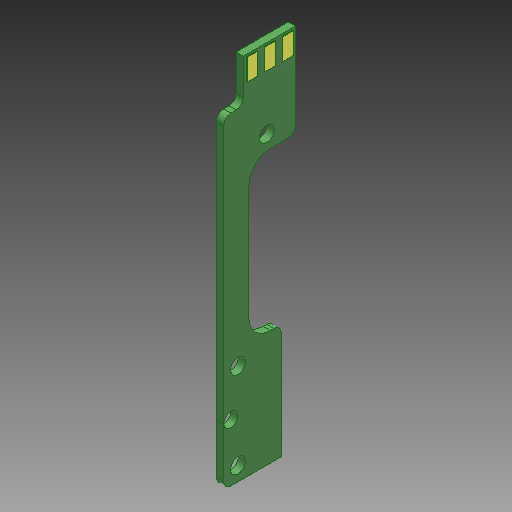
# Autodesk Inventor part: IR Platine
Saved by Autodesk Inventor 2019.1 (Build 231200000, 200)
## iProperties
Part Number: IR Platine
Material: Phenolharz
Document SubType Name: Modeling
Designer: rYan
Mass: 0.429024 g
Surface Area: 7.74127 cm^2
Volume: 0.310887 cm^3
Density: 1.38 g/cm^3
Appearance: Glatt - waldgrün
Author: rYan
Autodesk Inventor part; units mm, degrees
ref_plane "YZ Plane" through (0, 0, 0) normal (1, 0, 0) x (0, 1, 0)
ref_plane "XZ Plane" through (0, 0, 0) normal (0, 1, 0) x (-1, 0, 0)
ref_plane "XY Plane" through (0, 0, 0) normal (0, 0, 1) x (1, 0, 0)
sketch "Skizze1" plane through (0, 0, 0) normal (1, 0, 0) x (0, 1, 0)
  line L0 (0, 0) -> (8, 0)
  line L1 (8, 0) -> (8, 16)
  line L2 (8, 16) -> (3.5, 16)
  line L3 (0, 51) -> (0, 0)
  circle A0 centre (1, 8) radius 1
  circle A1 centre (2, 14) radius 1.05
  circle A2 centre (2, 2) radius 1.05
  line L4 (2, 14) -> (2, 2) construction
  line L5 (2, 8) -> (1, 8) construction
  line L6 (3.5, 16) -> (3.5, 38)
  line L7 (3.5, 38) -> (10, 38)
  line L8 (10, 38) -> (10, 51)
  line L9 (10, 51) -> (0, 51)
  dimension "d1" = 16
  dimension "d2" = 2
  dimension "d3" = 1
  dimension "d4" = 8
  dimension "d5" = 2.1
  dimension "d6" = 2.1
  dimension "d14" = 12
  dimension "d15" = 1
  dimension "d28" = 8
  dimension "d29" = 3.5
  dimension "d30" = 35
  dimension "d31" = 10
  dimension "d32" = 13
  constraints: 20 end point, 3 centre point, 3 horizontal, 3 parallel, 2 perpendicular, 1 midpoint, 1 vertical
  measures "d1" distance of L1.end L0.end
  measures "d2" diameter of A0
  measures "d3" distance from line of L5.end L3
  measures "d4" distance from line of L5.end L0
  measures "d5" diameter of A1
  measures "d6" diameter of A2
  measures "d14" distance of L4.start L4.end
  measures "d15" distance of L5.start L5.end
  measures "d28" distance between parallel lines of L3 L1
  measures "d29" distance between parallel lines of L3 L6
  measures "d30" distance between parallel lines of L2 L9
  measures "d31" distance of L8.end L3.start
  measures "d32" distance between parallel lines of L9 L7
extrude "Extrusion1" add sketch "Skizze1" along normal blind 1
sketch "Skizze2" plane through (0, 0, 0) normal (-1, 0, 0) x (0, 0, 1)
  circle A0 centre (2, 2) radius 1.05 projected
  circle A1 centre (14, 2) radius 1.05 projected
  line L0 (0, 0) -> (0, 8) projected
  line L1 (8, 0) -> (0, 0) projected
  circle A2 centre (8, 1) radius 1 projected
  line L2 (51, 0) -> (8, 0) projected
  line L3 (16, 8) -> (16, 3.5) projected
  line L4 (0, 8) -> (16, 8) projected
  line L5 (50.7, 3.15) -> (47.7, 3.15)
  line L6 (47.7, 3.15) -> (47.7, 4.65)
  line L7 (47.7, 4.65) -> (50.7, 4.65)
  line L8 (50.7, 4.65) -> (50.7, 3.15)
  line L9 (50.7, 5.65) -> (47.7, 5.65)
  line L10 (47.7, 5.65) -> (47.7, 7.15)
  line L11 (47.7, 7.15) -> (50.7, 7.15)
  line L12 (50.7, 7.15) -> (50.7, 5.65)
  line L13 (50.7, 8.15) -> (47.7, 8.15)
  line L14 (47.7, 8.15) -> (47.7, 9.65)
  line L15 (47.7, 9.65) -> (50.7, 9.65)
  line L16 (50.7, 9.65) -> (50.7, 8.15)
  line L17 (51, 10) -> (51, 0) projected
  line L18 (38, 10) -> (51, 10) projected
  line L19 (38, 3.5) -> (38, 10) projected
  line L20 (16, 3.5) -> (38, 3.5) projected
  line L21 (50.7, 3.9) -> (47.7, 3.9) construction
  line L22 (47.7, 6.4) -> (50.7, 6.4) construction
  line L23 (50.7, 8.9) -> (47.7, 8.9) construction
  dimension "d16" = 1.5
  dimension "d17" = 1.5
  dimension "d21" = 3
  dimension "d26" = 1.5
  dimension "d34" = 2.5
  dimension "d35" = 2.5
  dimension "d36" = 0.3
  dimension "d37" = 6.4
  constraints: 30 end point, 6 midpoint, 6 parallel, 3 horizontal, 3 perpendicular, 2 collinear, 2 point on line, 1 vertical alignment
  measures "d16" distance of L5.end L6.end
  measures "d17" distance of L9.end L10.end
  measures "d21" distance of L10.end L11.end
  measures "d26" distance of L13.end L14.end
  measures "d34" distance between parallel lines of L22 L21
  measures "d35" distance between parallel lines of L23 L22
  measures "d36" distance between parallel lines of L17 L12
  measures "d37" distance between parallel lines of L2 L22
extrude "Extrusion2" add sketch "Skizze2" along normal blind 0.1 and the other way blind 1.1 contours L5 L6 L7 L8 | L9 L10 L11 L12 | L13 L14 L15 L16
fillet "Rundung1" radius 3 2 edges at (0.5, 3.5, 16) (0.5, 3.5, 38)
sketch "Skizze3" plane through (0, 0, 51) normal (-1, 0, 0) x (0, 0, 1)
  circle A0 centre (-43, 1) radius 1 projected
  point P0 (-51, 0)
  point P1 (-11, 6)
  point P2 (-43, 0)
  dimension "d38" = 5
  dimension "d39" = 32
  constraints: 1 vertical alignment
  measures "d38" vertical distance of point (-11, 6) point (-43, 1)
  measures "d39" horizontal distance of point (-43, 1) point (-11, 6)
hole "Bohrung1" at (0, 6, 40) direction (1, 0, 0) diameter 2.1 end through all
fillet "Rundung2" radius 1 2 edges at (0.5, 10, 38) (0.5, 8, 16)
fillet "Rundung3" radius 1 1 edges at (0.5, 0, 0)
sketch "Skizze4" plane through (1, 1, 8) normal (1, 0, 0) x (0, 0, -1)
  line L0 (-43, -1) -> (0, -1) projected
  line L1 (-43, 9) -> (-43, -1) projected
  line L2 (-43, -1) -> (-37, -1)
  line L3 (-37, -1) -> (-37, 1.75)
  line L4 (-37, 1.75) -> (-43, 1.75)
  line L5 (-43, 1.75) -> (-43, -1)
  point P0 (8, -1)
  dimension "d52" = 2.75
  dimension "d53" = 6
  constraints: 8 end point, 2 parallel, 1 horizontal, 1 perpendicular
  measures "d52" distance of L2.end L3.end
  measures "d53" distance of L3.end L4.end
extrude "Extrusion3" cut sketch "Skizze4" against normal through all
fillet "Rundung4" radius 1 2 edges at (0.5, 2.75, 45) (0.5, 0, 45)
